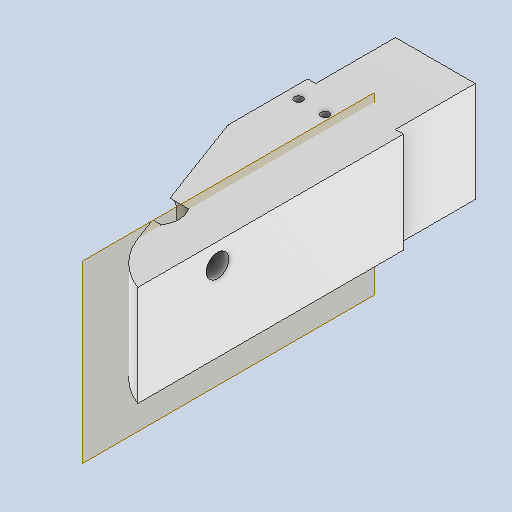
# Autodesk Inventor part: MontageAufnahmeLO
Saved by Autodesk Inventor 2025 (Build 290162010, 162A)
## iProperties
Created: 2024-11-18
Part Number: MontageAufnahmeLO
Material: PC/ABS-Kunststoff, 3DDruck, PLA
Document SubType Name: Modeling
Designer: Admin
Density: 1.1 g/cm^3
Appearance: Glatt - Weiß(2)
Mass: 29.2248 g
Surface Area: 64.7654 cm^2
Volume: 26.568 cm^3
Author: Admin
Autodesk Inventor part; units mm, degrees
ref_plane "YZ Plane" through (0, 0, 0) normal (1, 0, 0) x (0, 1, 0)
ref_plane "XZ Plane" through (0, 0, 0) normal (0, 1, 0) x (-1, 0, 0)
ref_plane "XY Plane" through (0, 0, 0) normal (0, 0, 1) x (1, 0, 0)
sketch "Skizze1" plane through (0, 0, 0) normal (0, 0, 1) x (1, 0, 0)
  line L0 (-9, -11.731) -> (9, -11.731) construction
  arc A0 (1.0455, -69.7765) -> (9, -77.731) centre (13.7004, -65.076) ccw
  line L1 (1.0455, -69.7765) -> (9, -69.7765) construction
  line L2 (9, -77.731) -> (9, -69.7765)
  line L3 (9, -77.731) -> (4, -77.731) construction
  line L4 (9, -27.731) -> (9, -69.7765)
  line L5 (-9, -42.731) -> (1.0455, -69.7765)
  line L6 (7.5, -10.731) -> (-7.5, -10.731) projected
  line L7 (-7.5, -10.731) -> (-7.5, 4.269) projected
  line L8 (-7.5, 4.269) -> (-9, 4.269) projected
  line L9 (-9, 4.269) -> (-9, -27.731) projected
  line L10 (-9, -27.731) -> (-7.5, -27.731) projected
  line L11 (-7.5, -27.731) -> (-7.5, -12.731) projected
  line L12 (-7.5, -12.731) -> (7.5, -12.731) projected
  line L13 (7.5, -12.731) -> (7.5, -27.731) projected
  line L14 (7.5, -27.731) -> (9, -27.731) projected
  line L15 (9, -27.731) -> (9, 4.269) projected
  line L16 (9, 4.269) -> (7.5, 4.269) projected
  line L17 (7.5, 4.269) -> (7.5, -10.731) projected
  line L18 (-9, -27.731) -> (-9, -42.731)
  point P0 (0, 0)
  dimension "d0" = 5
  dimension "d1" = 50
  dimension "d4" = 15
  constraints: 14 end point, 2 midpoint, 2 perpendicular, 2 point on circle, 2 vertical, 1 centre point, 1 coincident, 1 collinear, 1 horizontal, 1 point on line, 1 tangent
  measures "d0" distance of L3.start L3.end
  measures "d1" distance of L4.start L3.start
  measures "d4" distance of L9.end L5.start
extrude "Extrusion1" add sketch "Skizze1" against normal blind 18.9195 contours L5 L18 L10 L11 L12 L13 L14 L4 L2 A0
sketch "Skizze3" plane through (0, 0, 0) normal (0, 0, 1) x (1, 0, 0)
  circle A0 centre (-13.05, -31.8813) radius 1.621 construction
  line L0 (-13.05, -31.8813) -> (-6.55, -31.8813) construction
  line L1 (-6.55, -31.8813) -> (-1.55, -31.8813) construction
  point P0 (0, 0)
  dimension "d14" = 6.5
  dimension "d15" = 5
  constraints: 4 coincident, 4 end point, 1 horizontal, 1 point on line
  measures "d14" distance of L0.start L0.end
  measures "d15" distance of L0.end L1.end
hole "Bohrung2" at (-6.55, -31.8813, 0) at (-1.55, -31.8813, 0) direction (0, 0, -1) diameter 1.567 depth 10 tip angle 118 thread size "M2x0.4" class "6H" standard "ANSI Metric M Profile"
sketch "Skizze4" plane through (-7.5, -27.731, 0) normal (-1, 0, 0) x (0, 0, 1)
  circle A0 centre (-23.004, 8.5) radius 2.5 projected
  point P0 (0, 27.731)
hole "Bohrung3" at (-7.5, -19.231, -23.004) direction (1, 0, 0) diameter 5.3 end through all clearance for "Flachkopfmaschinenschraube" size "M5" standard "ANSI Metrisches M Profil"
ref_plane "Arbeitsebene1" through (1, -77.731, 0) normal (1, 0, 0) x (0, 0, -1)
sketch "Skizze5" plane through (1, -77.731, 0) normal (1, 0, 0) x (0, 0, -1)
  line L0 (18.9195, 50) -> (18.9195, 0) projected
  point P0 (0, 77.731)
  point P1 (3.9195, 15)
  dimension "d31" = 15
  dimension "d32" = 15
  measures "d31" distance from line of L0 point (3.919, 15)
  measures "d32" horizontal distance of L0.end point (3.919, 15)
hole "Bohrung4" at (1, -62.731, -3.9195) direction (1, 0, 0) diameter 4.3 end through all start extended yes countersink diameter 9.4 countersink angle 90 clearance for "Flachkopfmaschinenschraube" size "M4" standard "ANSI Metrisches M Profil"
